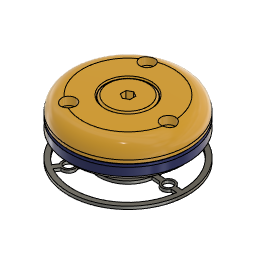
Bowden_Guide_360_Joint_20mm (Autodesk Fusion 360 design; units mm, degrees)
Autodesk Fusion 360 part; units mm, degrees
sketch "Skizze1" plane through (0, 0, 0) normal (0, 0, 1) x (1, 0, 0)
  circle A0 centre (0, 0) radius 25
  dimension "d1" = 50
  constraint coincident A0.centre origin
  measures "d1" diameter of A0
extrude "Extrusion1" add sketch "Skizze1" along normal blind 8 makes body 1
ref_plane "Arbeitsebene1" through (0, 0, 8) normal (0, 0, 1) x (1, 0, 0)
extrude "Extrusion2" add 1 faces at (-6.7759, -1.242, 0) along direction (0, 0, -1) blind 6 separate body on bodies 1 makes body 2
chamfer "Fase5" distance 2 angle 45 1 edges at (-23.3082, 9.0404, -6) on bodies 2
sketch "Skizze6" plane through (0, 0, 8) normal (0, 0, 1) x (-1, 0, 0)
  line L0 (0, 0) -> (14, -28) construction
  line L1 (0, 0) -> (-31.6764, 1.9013) construction
  line L2 (0, 0) -> (16.2848, 24.6645) construction
  circle A0 centre (9.9178, 15.0212) radius 1.75
  circle A1 centre (8.0498, -16.0997) radius 1.75
  circle A2 centre (-18, 1.0804) radius 1.75
  circle A3 centre (-18, 1.0804) radius 3
  circle A4 centre (8.0498, -16.0997) radius 3
  circle A5 centre (9.9178, 15.0212) radius 3
  circle A6 centre (0, 0) radius 25
  dimension "d19" = 120
  dimension "d20" = 120
  dimension "d21" = 3.5
  dimension "d22" = 3.5
  dimension "d23" = 3.5
  dimension "d24" = 18
  dimension "d25" = 18
  dimension "d26" = 18
  dimension "d29" = 6
  dimension "d30" = 6
  dimension "d31" = 6
  constraint coincident L0.start L1.start
  constraint coincident L2 A0.centre
  constraint coincident L0 A1.centre
  constraint coincident L1 A2.centre
  constraint concentric A2 A3
  constraint concentric A1 A4
  constraint concentric A0 A5
  measures "d19" angle of L0 L2
  measures "d20" angle of L0 L1
  measures "d21" diameter of A0
  measures "d22" diameter of A1
  measures "d23" diameter of A2
  measures "d24" horizontal distance of L0.start A2.centre
  measures "d25" distance of L0.start A1.centre
  measures "d26" distance of L0.start A0.centre
  measures "d29" diameter of A3
  measures "d30" diameter of A4
  measures "d31" diameter of A5
extrude "Extrusion5" cut sketch "Skizze6" against normal blind 4 contours A0 | A1 | A2 | A3 | A4 | A5 bodies 1
extrude "Extrusion6" cut sketch "Skizze6" against normal blind 15 contours A0 | A1 | A2 bodies 1 2
chamfer "Fase6" distance 0.6 angle 45 3 edges at (-7.1208, -16.1061, 4) (20.797, -2.1653, 4) (-5.2529, 15.0148, 4) on bodies 1
ref_plane "Arbeitsebene2" through (0, 0, -2) normal (0, 0, -1) x (-1, 0, 0)
ref_plane "Arbeitsebene3" through (0, 0, 4) normal (0, 0, 1) x (1, 0, 0)
sphere "Grundkörper Kugel4" cut diameter 20 placed x (1, 0, 0) y (0, 1, 0) z (0, 0, 1) at (0, 0, 4) bodies 1
sphere "Grundkörper Kugel5" add diameter 19.75 placed x (1, 0, 0) y (0, 1, 0) z (0, 0, 1) at (0, 0, 4) separate body makes body 3
fillet "Abrundung2" radius 6 1 edges at (-23.3082, -9.0404, 8) on bodies 1
ref_plane "Arbeitsebene4" through (-0.2974, -0.0964, 8) normal (0, 0, 1) x (1, 0, 0)
split "Teilen3" by plane through (-0.2974, -0.0964, 8) normal (0, 0, 1) bodies 3 makes body 4 at (7.4036, 1.3055, 10.403)
ref_plane "Arbeitsebene5" through (0, 0, 0) normal (0, 0, -1) x (-1, 0, 0)
split "Teilen4" by plane through (0, 0, 0) normal (0, 0, -1) bodies 3 makes body 5 at (7.4036, 1.3055, -2.403)
sketch "Skizze10" plane through (0, 0, 8) normal (0, 0, 1) x (-1, 0, 0)
  circle A0 centre (0, 0) radius 9.0286
  circle A1 centre (0, 0) radius 2.375 construction
  line L0 (0, 2.5) -> (0, -2.5) construction
  line L1 (0, 0) -> (2.0568, 1.1875) construction
  line L2 (0, 0) -> (-2.0568, 1.1875) construction
  line L3 (0, 0) -> (0.2151, 0)
  line L4 (0, 0) -> (-2.476, -1.4295) construction
  line L5 (0, 2.375) -> (-2.0568, 1.1875)
  line L6 (0, 2.375) -> (2.0568, 1.1875)
  line L7 (-2.0568, 1.1875) -> (-2.0568, -1.1875)
  line L8 (0, 0) -> (2.9692, -1.7143) construction
  line L9 (-2.0568, -1.1875) -> (0, -2.375)
  line L10 (2.0568, -1.1875) -> (0, -2.375)
  line L11 (2.0568, -1.1875) -> (2.0568, 1.1875)
  dimension "d46" = 4.75
  dimension "d47" = 60
  dimension "d48" = 60
  dimension "d49" = 60
  dimension "d50" = 60
  constraint concentric A0 A1
  constraint vertical L0
  constraint coincident A0.centre A1.centre
  constraint coincident A1 L1.end
  constraint coincident A1 L2.end
  constraint perpendicular L0 L3
  constraint coincident A1 L5.start
  constraint coincident L0 L5.start
  constraint coincident A1 L7.end
  constraint coincident L4 L7.end
  constraint coincident L0 L9.end
  constraint coincident A1 L9.end
  constraint coincident A1 L10.start
  constraint coincident L8 L10.start
  measures "d46" diameter of A1
  measures "d47" angle of L0 L2
  measures "d48" angle of L0 L1
  measures "d49" angle of L2 L4
  measures "d50" angle of L1 L8
extrude "Extrusion7" cut sketch "Skizze10" against normal blind 20 contours L5 L6 L7 L9 L10 L11 bodies 3
chamfer "Fase7" distance 0.64 angle 45 1 edges at (3.2649, 8.4176, 0) on bodies 3
chamfer "Fase8" distance 0.64 angle 45 1 edges at (3.2649, -8.4176, 8) on bodies 3
chamfer "Fase9" distance 0.64 angle 45 1 edges at (-3.3143, -8.5449, 8) on bodies 1
chamfer "Fase10" distance 0.64 angle 45 1 edges at (-3.3143, 8.5449, 0) on bodies 1
sketch "Skizze11" plane through (0, 0, 0) normal (0, 0, -1) x (1, 0, 0)
  circle A0 centre (0, 0) radius 25
  circle A1 centre (-8.0498, -16.0997) radius 1.75
  circle A2 centre (-9.9178, 15.0212) radius 1.75
  circle A3 centre (18, 1.0804) radius 1.75
  circle A4 centre (0, 0) radius 9.8052
  line L0 (-10, 0) -> (-7.1375, 0)
  line L1 (-7.1375, 0) -> (-7.1375, -0.2039)
  line L2 (-7.1375, -0.2039) -> (-10, -0.2039)
  line L3 (-10, -0.2039) -> (-10, 0)
  constraint horizontal L0
  constraint vertical L1
  constraint horizontal L2
  constraint vertical L3
extrude "Extrusion8" add sketch "Skizze11" against normal blind 0.05 contours A4 L0 L1 L2 | A4 L0 L2 L3 picked at (-8.0264, -0.1133) bodies 1 3
chamfer "Fase11" distance 0.64 angle 45 6 edges at (-1.0284, -1.7812, 0) (-2.0568, 0, 0) (-1.0284, 1.7812, 0) (1.0284, 1.7812, 0) (2.0568, 0, 0) (1.0284, -1.7812, 0) on bodies 1
chamfer "Fase12" distance 0.64 angle 45 3 edges at (19.6316, -0.4476, 0) (-6.4183, 16.7325, 0) (-8.2862, -14.3884, 0) on bodies 1
sketch "Skizze13" plane through (0, 0, -6) normal (0, 0, -1) x (1, 0, 0)
  circle A0 centre (18, 1.0804) radius 1.75
  circle A1 centre (-9.9178, 15.0212) radius 1.75
  circle A2 centre (-8.0498, -16.0997) radius 1.75
  circle A3 centre (0, 0) radius 23
  circle A4 centre (-9.9178, 15.0212) radius 2.25
  circle A5 centre (18, 1.0804) radius 2.25
  circle A6 centre (-8.0498, -16.0997) radius 2.25
  dimension "d61" = 4.5
  dimension "d62" = 4.5
  dimension "d63" = 4.5
  constraint concentric A1 A4
  constraint concentric A0 A5
  constraint concentric A2 A6
  measures "d61" diameter of A4
  measures "d62" diameter of A5
  measures "d63" diameter of A6
extrude "Extrusion9" cut sketch "Skizze13" against normal blind 4.2 contours A4 | A5 | A6 bodies 2
chamfer "Fase13" distance 0.64 angle 45 1 edges at (-23.3082, -9.0404, 0) on bodies 2
chamfer "Fase14" distance 0.64 angle 45 3 edges at (-8.2862, -15.654, 0) (19.6316, -1.7132, 0) (-6.4183, 15.4669, 0) on bodies 2
chamfer "Fase15" distance 0.64 angle 45 1 edges at (-23.3082, -9.0404, 0) on bodies 1
sketch "Skizze14" plane through (0, 0, 0) normal (0, 0, 1) x (-1, 0, 0)
  circle A0 centre (0, 0) radius 25
  line L0 (13.5006, 18.6223) -> (12.1676, 16.606)
  line L1 (11.7402, 19.7779) -> (10.4002, 17.727)
  arc A1 (11.7402, 19.7779) -> (-22.8638, 2.4992) centre (0, 0) ccw
  line L2 (-22.8638, 2.4992) -> (-20.4429, 2.3432)
  line L3 (-22.9981, 0.3796) -> (-20.6173, 0.2366)
  line L4 (11.2778, -20.0467) -> (10.1732, -17.8583)
  line L5 (9.2999, -21.0373) -> (8.2094, -18.841)
  arc A2 (-22.9981, 0.3796) -> (9.2999, -21.0373) centre (0, 0) ccw
  arc A3 (11.2778, -20.0467) -> (13.5006, 18.6223) centre (0, 0) ccw
  circle A4 centre (0, 0) radius 1.75
  circle A5 centre (9.9217, 15.019) radius 2
  circle A6 centre (8.0629, -16.095) radius 2
  line L6 (7.7214, -13.3662) -> (6.1905, -10.2799)
  line L7 (5.5215, -8.931) -> (1.8977, -1.6253)
  line L8 (5.9561, -14.3275) -> (4.3984, -11.1648)
  line L9 (3.7331, -9.814) -> (0.1294, -2.4966)
  line L10 (9.3411, 12.331) -> (7.4225, 9.429)
  line L11 (6.592, 8.1729) -> (2.0919, 1.3664)
  line L12 (7.6339, 13.493) -> (5.7129, 10.5529)
  line L13 (4.8892, 9.2922) -> (0.4265, 2.4619)
  arc A7 (4.8892, 9.2922) -> (-10.3625, 1.6934) centre (0, 0) ccw
  arc A8 (5.7129, 10.5529) -> (-11.8657, 1.7903) centre (0, 0) ccw
  line L14 (-15.4152, 2.0191) -> (-11.8657, 1.7903)
  line L15 (-10.3625, 1.6934) -> (-2.2088, 1.1679)
  line L16 (-15.5025, -0.0706) -> (-11.9967, -0.2812)
  line L17 (-10.4934, -0.3716) -> (-2.3471, -0.8609)
  arc A9 (-10.4934, -0.3716) -> (3.7331, -9.814) centre (0, 0) ccw
  arc A10 (5.5215, -8.931) -> (6.592, 8.1729) centre (0, 0) ccw
  arc A11 (-11.9967, -0.2812) -> (4.3984, -11.1648) centre (0, 0) ccw
  arc A12 (6.1905, -10.2799) -> (7.4225, 9.429) centre (0, 0) ccw
  circle A13 centre (-18, 1.0804) radius 2
  arc A14 (-20.6173, 0.2366) -> (-15.5025, -0.0706) centre (-18, 1.0804) ccw
  arc A15 (-15.4152, 2.0191) -> (-20.4429, 2.3432) centre (-18, 1.0804) ccw
  arc A16 (9.3411, 12.331) -> (12.1676, 16.606) centre (9.9217, 15.019) ccw
  arc A17 (10.4002, 17.727) -> (7.6339, 13.493) centre (9.9217, 15.019) ccw
  arc A18 (5.9561, -14.3275) -> (8.2094, -18.841) centre (8.0629, -16.095) ccw
  arc A19 (10.1732, -17.8583) -> (7.7214, -13.3662) centre (8.0629, -16.095) ccw
  arc A20 (-2.3471, -0.8609) -> (0.1294, -2.4966) centre (0, 0) ccw
  arc A21 (1.8977, -1.6253) -> (2.0919, 1.3664) centre (0, 0) ccw
  arc A22 (0.4265, 2.4619) -> (-2.2088, 1.1679) centre (0, 0) ccw
  dimension "d75" = 46
  dimension "d84" = 3.5
  dimension "d85" = 4
  dimension "d86" = 4
  dimension "d87" = 24
  dimension "d88" = 21
  dimension "d89" = 5.5
  dimension "d90" = 4
  dimension "d91" = 5.5
  dimension "d92" = 5.5
  dimension "d93" = 5
  constraint collinear L0 L10
  constraint collinear L1 L12
  constraint concentric A1 A2
  constraint collinear L2 L14
  constraint collinear L3 L16
  constraint coincident L4.start A2
  constraint concentric A2 A3
  constraint concentric A1 A8
  constraint coincident L6.end A8
  constraint coincident L7.start A7
  constraint collinear L6 L7
  constraint coincident L8.end A8
  constraint coincident L9.start A7
  constraint collinear L8 L9
  constraint collinear L10 L11
  constraint collinear L12 L13
  constraint coincident A7.end L14
  constraint coincident L17.start L16
  constraint concentric A7 A9
  constraint concentric A8 A11
  constraint collinear L14 L15
  constraint collinear L16 L17
  constraint concentric A9 A10
  constraint concentric A11 A12
  constraint coincident L14.start A14
  constraint concentric A14 A15
  constraint concentric A5 A16
  constraint coincident L1.end A16
  constraint concentric A16 A17
  constraint concentric A6 A18
  constraint coincident L4.end A18
  constraint concentric A18 A19
  constraint concentric A3 A20
  constraint concentric A20 A21
  constraint coincident L13.end A21
  constraint concentric A21 A22
  measures "d75" diameter of A1
  measures "d84" diameter of A4
  measures "d85" diameter of A5
  measures "d86" diameter of A6
  measures "d87" diameter of A8
  measures "d88" diameter of A7
  measures "d89" diameter of A14
  measures "d90" diameter of A13
  measures "d91" diameter of A16
  measures "d92" diameter of A18
  measures "d93" diameter of A20
extrude "Extrusion10" add sketch "Skizze14" along normal blind 1.2 separate body makes body 6
sketch "Skizze15" plane through (0, 0, -6) normal (0, 0, -1) x (1, 0, 0)
  circle A0 centre (18, 1.0804) radius 2.25
  circle A1 centre (-8.0498, -16.0997) radius 2.25
  circle A2 centre (0, 0) radius 23
  circle A3 centre (0, 0) radius 10
  circle A4 centre (-9.9178, 15.0212) radius 2.25
  dimension "d94" = 20
  constraint coincident A2.centre A3.centre
  measures "d94" diameter of A3
extrude "Extrusion11" cut sketch "Skizze15" against normal blind 6 contours A3 bodies 2
chamfer "Fase18" distance 4 distance2 6 1 edges at (-9.3233, -3.6162, -6) measured on face at (14.7136, -7.2062, -6) on bodies 2
move_body "Move1" bodies 6 to x (1, 0, 0) y (0, 1, 0) z (0, 0, 1) at (0, 0, -16)
hidden bodies 4 5
named bodies: "Top_20mm", "Bottom_20mm", "Drill_Guide"
